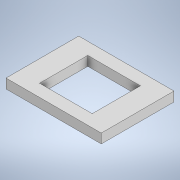
# Autodesk Inventor part: RoadBot Pneumatic Module - Connection Bay Cover- r2
Saved by Autodesk Inventor 2020 (Build 240168000, 168)
## iProperties
Created: 2022-04-02
Part Number: RoadBot Pneumatic Module - Connection Bay Cover- r2
Material: Generic
Document SubType Name: Modeling
Designer: Beaucage
Density: 1 g/cm^3
Appearance: Default
Author: Beaucage
Autodesk Inventor part; units mm, degrees
ref_plane "YZ Plane" through (0, 0, 0) normal (1, 0, 0) x (0, 1, 0)
ref_plane "XZ Plane" through (0, 0, 0) normal (0, 1, 0) x (-1, 0, 0)
ref_plane "XY Plane" through (0, 0, 0) normal (0, 0, 1) x (1, 0, 0)
sketch "Sketch1" plane through (0, 0, 0) normal (0, 1, 0) x (-1, 0, 0)
  line L0 (0, 0) -> (31.9786, 0)
  line L1 (31.9786, 0) -> (31.9786, -24.4094)
  line L2 (31.9786, -24.4094) -> (0, -24.4094)
  line L3 (0, -24.4094) -> (0, 0)
  dimension "d0" = 31.9786
  dimension "d1" = 24.4094
  constraints: 8 end point, 2 parallel, 1 horizontal, 1 perpendicular
  measures "d0" distance of L1.end L2.end
  measures "d1" distance of L0.end L1.end
extrude "Extrusion1" add sketch "Sketch1" along normal blind 3.175
sketch "Sketch2" plane through (0, 3.175, 0) normal (0, 1, 0) x (1, 0, 0)
  line L0 (-31.9786, 24.4094) -> (-31.9786, 0) projected
  line L1 (-31.9786, 12.2047) -> (0, 12.2047)
  line L2 (0, 0) -> (0, 24.4094) projected
  line L3 (-24.8332, 4.1101) -> (-7.1454, 4.1101)
  line L4 (-7.1454, 4.1101) -> (-7.1454, 20.2993)
  line L5 (-7.1454, 20.2993) -> (-24.8332, 20.2993)
  line L6 (-24.8332, 20.2993) -> (-24.8332, 4.1101)
  line L7 (-24.8332, 4.1101) -> (-7.1454, 20.2993) construction
  line L8 (-7.1454, 4.1101) -> (-24.8332, 20.2993) construction
  point P0 (-15.9893, 12.2047)
  dimension "d4" = 17.6878
  dimension "d5" = 16.1892
  constraints: 14 end point, 5 midpoint, 2 parallel, 1 horizontal, 1 perpendicular
  measures "d4" distance of L5.end L4.end
  measures "d5" distance of L4.end L3.end
extrude "Extrusion2" cut sketch "Sketch2" against normal blind 25.4
body "Solid1"
